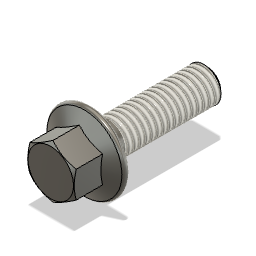
Motor_Mount v2 (Autodesk Fusion 360 archive; units mm, degrees)
design "Hex Flange Screw ANSI B18.2.3.4M - M6 x 1x20 Steel Grade 2 Plain"
description: Hex Flange Screw ANSI B18.2.3.4M - M6 x 1x20
Autodesk Fusion 360 part; units mm, degrees
sketch "Sketch1" plane through (0, 0, 0) normal (0, 1, 0) x (1, 0, 0)
  line L0 (-3, 0) -> (-3, 20)
  line L1 (-3, 20) -> (0, 20)
  line L2 (0, 20) -> (0, -6.9)
  line L3 (-3, 0) -> (-4.62, 0)
  line L4 (-4.62, 0) -> (-4.62, -6.4959)
  line L5 (-3.92, -6.9) -> (0, -6.9)
  line L6 (-3.92, -6.9) -> (-4.62, -6.4959)
  dimension "d9" = 6
  dimension "d68" = 20
  dimension "d111" = 6.9
  dimension "d114" = 9.24
  dimension "d115" = 7.84
  dimension "d159" = 30
  constraint perpendicular L0 L1
  constraint perpendicular L0 L3
  constraint coincident origin L3
  constraint vertical L0
  constraint vertical L2
  constraint parallel L2 L4
  constraint coincident L2 L5.end
  constraint perpendicular L2 L5
  constraint coincident L3.end L4.start
  constraint coincident origin L2
  measures "d68" distance of origin L1.end
  measures "d111" distance of L3 L5
  measures "d159" angle of L5 L6
revolve "Revolve1" add sketch "Sketch1" angle 360 about axis through (0, 0, -20) along (0, 0, 1)
sketch "Sketch8" plane through (0, 0, 6.9) normal (0, 0, 1) x (1, 0, 0)
  line L0 (-4, -2.3118) -> (-4, 2.3118)
  circle A0 centre (0, 0) radius 3.92
  circle A1 centre (0, 0) radius 4.62
  dimension "d110" = 4
  constraint coincident L0.end A1
  constraint coincident L0.start A1
  constraint vertical L0
  measures "d110" distance of A0.centre L0
extrude "Extrude5" cut sketch "Sketch8" against normal blind 6.9 contours L0 A1 picked at (-4.1, 0.5631)
pattern_circular "C-Pattern2" count 6 over 360 about axis through (0, 0, 1.75) along (0, 0, 1) of "Extrude5"
sketch "Sketch12" plane through (0, 0, 0) normal (0, 1, 0) x (1, 0, 0)
  line L0 (3.8, 0) -> (6.223, 0)
  line L1 (6.4668, -1.1) -> (3.8, -2.3436)
  line L2 (3.8, -2.3436) -> (3.8, 0)
  arc A0 (6.4668, -1.1) -> (6.223, 0) centre (6.223, -0.577) ccw
  line L3 (0, -1.75) -> (0, -22.5)
  line L4 (4.62, 0) -> (4.62, -1.9612) construction
  line L5 (0, 0) -> (4, 0)
  line L6 (3.92, -6.9) -> (-3.92, -6.9)
  line L7 (6.223, -0.577) -> (6.8, -0.577) construction
  dimension "d122" = 7.6
  dimension "d126" = 9.24
  dimension "d138" = 1.1
  dimension "d161" = 25
  dimension "d162" = 6.8
  constraint horizontal L0
  constraint perpendicular L0 L2
  constraint tangent L0 A0
  constraint tangent L1 A0
  constraint horizontal L5.start L0.start
  constraint coincident L1 L4.end
  constraint perpendicular L0 L4
  constraint coincident L0 L4.start
  constraint coincident A0.centre L7.start
  constraint coincident A0 L7.end
  constraint horizontal L7
  measures "d138" vertical distance of L0.end L1.start
  measures "d161" angle of L0 L1
  measures "d162" horizontal distance of L5.start L7.end
revolve "Revolve3" add sketch "Sketch12" angle 360 about axis through (0, 0, 1.75) along (0, 0, 1)
fillet "Fillet4" radius 0.2 1 edges at (-2.797, 1.0848, 0)
thread "Thread2" "ISO Metric profile 6.0 M6x1 6g" major diameter 5.884 minor diameter 4.7435 pitch 1 angle 60 resizes the face on face at (-2.9963, 0.1495, -6.8) from (0, 0, -3) to (0, 0, -20)
sketch "Sketch5" plane through (0, 0, 0) normal (0, 1, 0) x (1, 0, 0)
  line L0 (-3.06, 20) -> (-3.06, 19.4)
  line L1 (-3.06, 19.4) -> (-2.4, 20)
  line L2 (0, 20) -> (0, -6.9)
  line L3 (-3.06, 20) -> (0, 20)
  dimension "d154" = 0.6
  dimension "d155" = 2.4
  dimension "d156" = 3.06
  constraint coincident L2.start L3.end
  constraint perpendicular L2 L3
  constraint coincident L1.end L3
  constraint perpendicular L0 L3
  measures "d154" vertical distance of L0.end L1.end
  measures "d155" horizontal distance of origin L1.end
  measures "d156" horizontal distance of origin L0.start
revolve "Revolve2" cut sketch "Sketch5" angle 360 about axis through (0, 0, -20) along (0, 0, 1)
equation "d9 = adsk_nomdia"
equation "adsk_nomlen = 20.00 mm"
equation "adsk_headh = 6.90 mm"
equation "adsk_nomdia = 6.00 mm"
equation "d68 = adsk_nomlen"
equation "d89 = -adsk_headh"
equation "adsk_waflat = 8.00 mm"
equation "d110 = adsk_waflat / 2"
equation "d111 = adsk_headh"
equation "d114 = adsk_wacor"
equation "d115 = adsk_topdia"
equation "d122 = adsk_waflat * 0.95"
equation "d126 = adsk_waflat * 1.155"
equation "adsk_headdia = 13.60 mm"
equation "adsk_flngheig = 1.10 mm"
equation "adsk_thrlen = 17.00 mm"
equation "d133 = adsk_nomdia / 30"
equation "d138 = adsk_flngheig"
equation "d144 = min(adsk_thrlen; adsk_nomlen - d133 - 0.01 mm)"
equation "adsk_endpointdia = adsk_nomdia - adsk_startlen * 2"
equation "adsk_startlen = 0.1 * adsk_nomdia"
equation "d154 = adsk_startlen"
equation "d155 = adsk_endpointdia / 2"
equation "d156 = adsk_nomdia * 0.51"
equation "adsk_chamang2 = 30 deg"
equation "adsk_flngang = 25 deg"
equation "d159 = adsk_chamang2"
equation "d161 = adsk_flngang"
equation "d162 = adsk_headdia / 2"
equation "adsk_topdia = adsk_waflat * 0.98"
equation "adsk_wacor = 9.24 mm"
